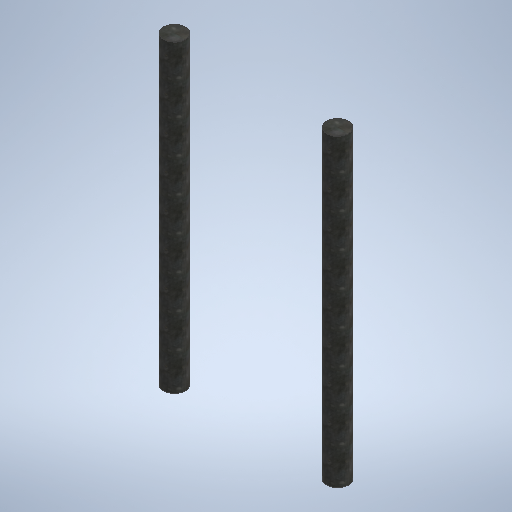
# Autodesk Inventor part: Cylinder Supports
Saved by Autodesk Inventor 2025 (Build 290162000, 162)
## iProperties
Created: 2024-06-26
Part Number: Cylinder Supports
Material: Steel ASTM A36
Document SubType Name: Modeling
Designer: track
Density: 7.85 g/cm^3
Appearance: Plate
Author: track
Autodesk Inventor part; units mm, degrees
ref_plane "YZ Plane" through (0, 0, 0) normal (1, 0, 0) x (0, 1, 0)
ref_plane "XZ Plane" through (0, 0, 0) normal (0, 1, 0) x (-1, 0, 0)
ref_plane "XY Plane" through (0, 0, 0) normal (0, 0, 1) x (1, 0, 0)
sketch "Sketch1" plane through (720.725, 0, -2101.85) normal (0, 1, 0) x (-1, 0, 0)
  line L0 (0, -25.4) -> (0, -88.9)
  line L1 (0, -57.15) -> (1266.7426, -57.15)
  circle A0 centre (533.4, -57.15) radius 57.15
  circle A1 centre (1384.3, -57.15) radius 57.15
  point P0 (984.25, 4318)
  dimension "d2" = 114.3
  dimension "d3" = 533.4
  dimension "d0" = 114.3
  dimension "d1" = 850.9
  constraints: 4 end point, 2 centre point, 2 point on line, 1 horizontal, 1 midpoint
  measures "d2" diameter of A0
  measures "d3" distance from line of L0 A0.centre
  measures "d0" diameter of A1
  measures "d1" distance of A0.centre A1.centre
extrude "Extrusion1" add sketch "Sketch1" along normal blind 1587.5
body "Solid1"
